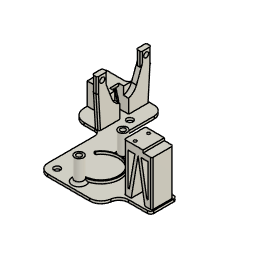
Uchyt na krokovy motor X (Autodesk Fusion 360 design; units mm, degrees)
Autodesk Fusion 360 part; units mm, degrees
sketch "Sketch1" plane through (0, 0, 0) normal (0, 0, 1) x (1, 0, 0)
  line L0 (25, 25) -> (25, -25)
  line L1 (25, -25) -> (-25, -25)
  line L2 (-25, -25) -> (-25, 25)
  circle A0 centre (0, 17.5) radius 2
  circle A1 centre (0, -17.5) radius 2
  line L3 (-48.5, 25) -> (-48.5, 65)
  line L4 (-48.5, 65) -> (-15, 65)
  line L5 (-15, 65) -> (-15, 25)
  line L6 (-25, 25) -> (-48.5, 25)
  line L7 (-15, 25) -> (25, 25)
  line L8 (-48.5, 37.5) -> (-30.5, 37.5)
  line L9 (-30.5, 37.5) -> (-30.5, 52.5)
  line L10 (-30.5, 52.5) -> (-48.5, 52.5)
  line L11 (-48.5, 52.5) -> (-48.5, 37.5)
  line L12 (-30.5, 41.5) -> (-34.5, 41.5)
  line L13 (-34.5, 41.5) -> (-34.5, 48.5)
  line L14 (-34.5, 48.5) -> (-30.5, 48.5)
  line L15 (-30.5, 48.5) -> (-30.5, 41.5)
  line L16 (-30.5, 25) -> (-34.5, 25)
  line L17 (-30.5, 65) -> (-34.5, 65)
  circle A2 centre (0, 17.5) radius 3.5
  circle A3 centre (0, -17.5) radius 3.5
  arc A4 (2.2613, -14.8286) -> (2.2613, 14.8286) centre (0, 0) ccw
  circle A5 centre (8, 0) radius 2.5
  circle A6 centre (-22, 45) radius 2.5
  line L18 (0, 7.5) -> (-12.9904, 7.5)
  line L19 (-12.9904, -7.5) -> (0, -7.5)
  arc A7 (-2.2613, 14.8286) -> (-12.9904, 7.5) centre (0, 0) ccw
  arc A8 (-12.9904, -7.5) -> (-2.2613, -14.8286) centre (0, 0) ccw
  arc A9 (-11.8216, -7.5) -> (-11.8216, 7.5) centre (0, 0) ccw
  dimension "d1" = 50
  dimension "d2" = 50
  dimension "d4" = 4
  dimension "d5" = 4
  dimension "d6" = 17.5
  dimension "d7" = 17.5
  dimension "d12" = 28
  dimension "d57" = 40
  dimension "d62" = 18
  dimension "d63" = 15
  dimension "d64" = 12.5
  dimension "d65" = 4
  dimension "d66" = 7
  dimension "d67" = 4
  dimension "d74" = 7
  dimension "d75" = 7
  dimension "d82" = 5
  dimension "d83" = 8
  dimension "d85" = 17.5
  dimension "d88" = 25
  dimension "d89" = 56.5
  dimension "d91" = 25
  dimension "d167" = 5
  dimension "d220" = 15
  dimension "d221" = 7.5
  constraint horizontal L6
  constraint vertical L0
  constraint horizontal L1
  constraint vertical L2
  constraint coincident A4.centre A7.centre
  constraint vertical L3
  constraint horizontal L4
  constraint vertical L5
  constraint coincident L5.end L6
  constraint collinear L6 L7
  constraint horizontal L8
  constraint vertical L9
  constraint horizontal L10
  constraint vertical L11
  constraint coincident L3 L8.start
  constraint horizontal L12
  constraint vertical L13
  constraint horizontal L14
  constraint vertical L15
  constraint coincident L9 L12.start
  constraint horizontal L16
  constraint coincident L6 L16.start
  constraint horizontal L17
  constraint coincident L4 L17.start
  constraint concentric A0 A2
  constraint coincident A2 A4.end
  constraint coincident A2 A7.start
  constraint concentric A1 A3
  constraint coincident A3 A8.end
  constraint coincident A3 A4.start
  constraint concentric A4 A7
  constraint horizontal L18
  constraint horizontal L19
  constraint concentric A7 A8
  constraint coincident L18 A9.end
  constraint coincident L19 A9.start
  measures "d1" distance of L2.end L0.start
  measures "d2" distance of L2.end L1.end
  measures "d4" diameter of A0
  measures "d5" diameter of A1
  measures "d6" distance of A4.centre A0.centre
  measures "d7" distance of A4.centre A1.centre
  measures "d12" diameter of A9
  measures "d57" distance of L3.start L3.end
  measures "d62" distance of L8.start L8.end
  measures "d63" distance of L8.end L9.end
  measures "d64" distance of L6 L8
  measures "d65" distance of L12.start L12.end
  measures "d66" distance of L12.end L13.end
  measures "d67" distance of L10 L14
  measures "d74" diameter of A2
  measures "d75" diameter of A3
  measures "d82" diameter of A5
  measures "d83" distance of A4.centre A5.centre
  measures "d85" vertical distance of A1.centre A5.centre
  measures "d88" distance of L2 A4.centre
  measures "d89" distance of L3 A5.centre
  measures "d91" vertical distance of L0.end A4.centre
  measures "d167" diameter of A6
  measures "d220" distance of L18.start L19.end
  measures "d221" distance of A4.centre L18
extrude "Extrude1" add sketch "Sketch1" along normal blind 22 contours A0 | A1 makes body 1 at (1.9975, -17.5997, 14.6667) makes body 2 at (1.9975, 17.4003, 14.6667)
extrude "Extrude2" add sketch "Sketch1" along normal blind 2 contours L0 L1 L2 L3 L4 L5 L6 L7 L8 L9 L10 L15 L16 L17 | L3 L8 L9 L10 L11 L12 L13 L14 | L9 L12 L13 L14 L15 | A2 | A2 L18 A7 A9 | A2 A3 A4 A9 | A3 | A3 L19 A8 A9 | A5 | A6 bodies 1 2
extrude "Extrude3" add sketch "Sketch1" along normal blind 4 contours A2 L18 A7 A9 | A2 A3 A4 A9 | A3 L19 A8 A9 bodies 1
extrude "Extrude4" add 2 faces at (0.1483, -18.0912, 22) (-0.1483, 17.7569, 22) along direction (0, 0, 1) blind 2 on bodies 1 bodies 1
fillet "Fillet1" radius 1 2 edges at (-1.8647, -18.2232, 24) (-1.8647, 16.7768, 24) on bodies 1
fillet "Fillet2" radius 0.5 3 edges at (-8.4605, -12.3863, 4) (15, 0, 4) (-8.4605, 12.3863, 4) on bodies 1
sketch "Sketch2" plane through (0, 0, 0) normal (0, 0, 1) x (1, 0, 0)
  line L0 (25, -10.5) -> (50, -10.5)
  line L1 (50, -10.5) -> (50, 10.5)
  line L2 (50, 10.5) -> (25, 10.5)
  line L3 (25, 10.5) -> (25, -10.5)
  line L4 (49, -8.5) -> (27, -8.5)
  line L5 (27, -8.5) -> (27, 8.5)
  line L6 (27, 8.5) -> (49, 8.5)
  line L7 (49, 8.5) -> (49, -8.5)
  dimension "d256" = 1
  constraint horizontal L0
  constraint vertical L1
  constraint horizontal L2
  constraint vertical L3
  constraint horizontal L4
  constraint vertical L5
  constraint horizontal L6
  constraint vertical L7
  measures "d21" distance of L4.start L4.end
  measures "d22" distance of L4.start L6.end
  measures "d23" distance of L0.start L0.end
  measures "d24" distance of L0.end L1.end
  measures "d25" distance of origin L0
  measures "d26" distance of L0 L4
  measures "d27" distance of L1 L7
extrude "Extrude5" add sketch "Sketch2" along normal blind 2 bodies 1
extrude "Extrude6" add sketch "Sketch2" along normal blind 40 contours L4 L5 L6 L7 bodies 1
sketch "Sketch3" plane through (0, 0, 40) normal (0, 0, 1) x (-1, 0, 0)
  line L0 (-49, -8.5) -> (-27, -8.5)
  line L1 (-27, -8.5) -> (-27, 8.5)
  line L2 (-27, 8.5) -> (-49, 8.5)
  line L3 (-49, 8.5) -> (-49, -8.5)
  line L4 (-49, 8.5) -> (-42, 8.5)
  line L5 (-42, 8.5) -> (-42, -8.5)
  line L6 (-42, -8.5) -> (-49, -8.5)
  line L7 (-49, -8.5) -> (-49, 8.5)
  dimension "d32" = 7
  constraint horizontal L4
  constraint vertical L5
  constraint horizontal L6
  constraint vertical L7
  constraint coincident L2.end L3.start
  measures "d32" distance of L2.end L4.end
extrude "Extrude7" cut sketch "Sketch3" against normal blind 2 contours L0 L2 L3 L4 L5 L6 L7 bodies 1
fillet "Fillet3" radius 1 4 edges at (27, 8.5, 21) (27, -8.5, 21) (49, -8.5, 20) (49, 8.5, 20) on bodies 1
sketch "Sketch4" plane through (0, 8.5, 0) normal (0, 1, 0) x (-1, 0, 0)
  line L0 (-48, 38) -> (-48, 2)
  line L1 (-48, 2) -> (-28, 2)
  line L2 (-28, 2) -> (-28, 40)
  line L3 (-28, 40) -> (-42, 40)
  line L4 (-42, 40) -> (-42, 38)
  line L5 (-42, 38) -> (-48, 38)
  line L6 (-43.4614, 2) -> (-38, 34)
  line L7 (-38, 34) -> (-32.538, 2)
  line L8 (-43.4614, 2) -> (-32.538, 2)
  line L9 (-45.9446, 34) -> (-40.5, 34)
  line L10 (-40.5, 34) -> (-44.9517, 7.9159)
  line L11 (-45.9446, 8) -> (-45.9446, 34)
  line L12 (-35.5, 34) -> (-30.0549, 34)
  line L13 (-30.0549, 34) -> (-30.0549, 8)
  line L14 (-31.0478, 7.9159) -> (-35.5, 34)
  arc A0 (-45.9446, 8) -> (-44.9517, 7.9159) centre (-45.4446, 8) ccw
  arc A1 (-31.0478, 7.9159) -> (-30.0549, 8) centre (-30.5549, 8) ccw
  dimension "d42" = 0.5
  dimension "d43" = 0.5
  dimension "d44" = 6
  dimension "d45" = 6
  dimension "d239" = 10
  dimension "d241" = 2.5
  dimension "d242" = 2.5
  dimension "d247" = 32
  dimension "d248" = 32
  dimension "d249" = 32
  constraint coincident L1 L6.start
  constraint coincident L1 L7.end
  constraint parallel L6 L10
  constraint perpendicular L9 L11
  constraint perpendicular L11 L12
  constraint perpendicular L12 L13
  constraint tangent L10 A0
  constraint tangent L11 A0
  constraint tangent L13 A1
  constraint tangent L14 A1
  constraint parallel L7 L14
  constraint parallel L8 L9
  measures "d42" radius of A0
  measures "d43" radius of A1
  measures "d44" distance of L8 A0.centre
  measures "d45" distance of L1 A1.centre
  measures "d239" distance of L2 L6.end
  measures "d241" horizontal distance of L6.end L9.end
  measures "d242" horizontal distance of L6.end L12.start
  measures "d247" distance of L8 L9
  measures "d248" distance of L8 L12
  measures "d249" distance of L6.end L8
extrude "Extrude8" cut sketch "Sketch4" against normal up to surface (17 mm away) contours L1 L6 L7 L8 bodies 1
extrude "Extrude9" cut sketch "Sketch4" against normal up to surface (17 mm away) contours L9 L10 L11 A0 | L12 L13 L14 A1 bodies 1
sketch "Sketch6" plane through (0, 0, 0) normal (0, 0, -1) x (1, 0, 0)
  line L0 (25, 25) -> (-25, 25)
  line L1 (-25, 25) -> (-25, -25)
  line L2 (-15, -25) -> (25, -25)
  line L3 (25, -25) -> (25, -10.5)
  circle A0 centre (38, 0) radius 2.5
  circle A1 centre (17.5, -17.5) radius 2.5
  line L4 (25, -25) -> (25, 25)
  circle A2 centre (-17.5, 17.5) radius 2.5
  line L5 (25, 25) -> (-25, 25)
  line L6 (-25, 25) -> (-25, -25)
  line L7 (-15, -65) -> (-15, -25)
  line L8 (-25, -25) -> (-48.5, -25)
  line L9 (-48.5, -25) -> (-48.5, -65)
  line L10 (-48.5, -65) -> (-15, -65)
  line L11 (-25, -25) -> (-48.5, -25)
  line L12 (25, -10.5) -> (50, -10.5)
  line L13 (50, -10.5) -> (50, 10.5)
  line L14 (50, 10.5) -> (25, 10.5)
  line L15 (25, 10.5) -> (25, 25)
  dimension "d46" = 5
  dimension "d47" = 5
  dimension "d48" = 7.5
  dimension "d50" = 5
  dimension "d51" = 7.5
  dimension "d52" = 7.5
  measures "d46" diameter of A0
  measures "d47" diameter of A1
  measures "d48" distance of A1.centre L4
  measures "d50" diameter of A2
  measures "d51" distance of A2.centre L5
  measures "d52" distance of A2.centre L6
extrude "Extrude10" cut sketch "Sketch6" against normal up to surface (2 mm away) contours A0 | A1 | A2 bodies 1
extrude "Extrude11" add sketch "Sketch1" along normal up to surface (4 mm away) contours A2 A3 A4 A9 bodies 1
extrude "Extrude12" add sketch "Sketch1" along normal blind 20 contours A2 | A3 bodies 1
extrude "Extrude13" cut sketch "Sketch1" along normal up to surface (24 mm away) contours A0 | A1 bodies 1
extrude "Extrude14" add sketch "Sketch1" along normal blind 18.5 contours L3 L8 L9 L10 L11 L12 L13 L14 bodies 1
extrude "Extrude15" add 1 faces at (-43.8333, 46.1667, 18.5) along direction (0, 0, 1) blind 2 on bodies 1 bodies 1
extrude "Extrude17" cut sketch "Sketch1" along normal blind 2 contours A6 bodies 1
sketch "Sketch7" plane through (-48.5, 0, 0) normal (-1, 0, 0) x (0, -1, 0)
  line L0 (-65, 0) -> (-25, 0)
  line L1 (-48.5, 2.5) -> (-45.3117, 17.5)
  line L2 (-45.3117, 17.5) -> (-44.6883, 17.5)
  line L3 (-44.6883, 17.5) -> (-41.5, 2.5)
  line L4 (-41.5, 2.5) -> (-48.5, 2.5)
  line L5 (-52.5, 20.5) -> (-52.5, 2)
  line L6 (-37.5, 2) -> (-37.5, 20.5)
  line L7 (-48.5, 17.5) -> (-46.334, 17.5)
  line L8 (-46.334, 17.5) -> (-48.5, 7.3097)
  line L9 (-48.5, 17.5) -> (-48.5, 7.3097)
  line L10 (-41.5, 17.5) -> (-43.666, 17.5)
  line L11 (-43.666, 17.5) -> (-41.5, 7.3097)
  line L12 (-41.5, 17.5) -> (-41.5, 7.3097)
  line L13 (-25, 2) -> (-37.5, 2)
  line L14 (-37.5, 20.5) -> (-52.5, 20.5)
  line L15 (-52.5, 2) -> (-65, 2)
  line L16 (-65, 2) -> (-65, 0)
  line L17 (-25, 0) -> (-25, 2)
  line L18 (-37.5, 2) -> (-37.5, 20.5)
  line L19 (-52.5, 20.5) -> (-52.5, 2)
  dimension "d142" = 78
  dimension "d143" = 78
  dimension "d144" = 4
  dimension "d145" = 4
  dimension "d147" = 4
  dimension "d149" = 1
  dimension "d150" = 78
  dimension "d152" = 1
  dimension "d153" = 4
  constraint perpendicular L7 L9
  measures "d142" angle of L3 L4
  measures "d143" angle of L1 L4
  measures "d144" distance of L1.start L5
  measures "d145" distance of L3.end L6
  measures "d147" distance of L5 L7.start
  measures "d149" distance of L1 L8.end
  measures "d150" angle of L7 L8
  measures "d152" distance of L3 L11
  measures "d153" distance of L6 L12
extrude "Extrude18" cut sketch "Sketch7" against normal up to surface (14 mm away) contours L1 L2 L3 L4 | L7 L8 L9 | L10 L11 L12 bodies 1
sketch "Sketch9" plane through (-30.5, 0, 0) normal (1, 0, 0) x (0, 1, 0)
  line L0 (37.5, 2) -> (41.5, 2)
  line L1 (41.5, 20.5) -> (37.5, 20.5)
  line L2 (25.1524, 0) -> (41.5, 0)
  line L3 (41.5, 0) -> (41.5, 13.0164)
  line L4 (23.5, 27.99) -> (23.5, 40)
  line L5 (23.5, 40) -> (31.5, 40)
  line L6 (31.5, 40) -> (31.5, 28.9965)
  line L7 (23.5, 27.99) -> (25.1524, 0)
  line L8 (37.5, 13.0164) -> (41.5, 13.0164)
  circle A0 centre (27.5, 36) radius 2
  line L9 (31.5, 28.9965) -> (37.5, 13.0164)
  line L10 (45, 2) -> (45, 38)
  line L11 (48.5, 0) -> (48.5, 13.0164)
  line L12 (58.5, 40) -> (58.5, 28.9965)
  line L13 (66.5, 40) -> (58.5, 40)
  line L14 (66.5, 27.99) -> (66.5, 40)
  circle A1 centre (62.5, 36) radius 2
  line L15 (66.5, 27.99) -> (64.8476, 0)
  line L16 (64.8476, 0) -> (48.5, 0)
  line L17 (41.5, 2) -> (41.5, 20.5)
  line L18 (48.5, 13.0164) -> (52.5, 13.0164)
  line L19 (52.5, 13.0164) -> (58.5, 28.9965)
  line L20 (52.5, 2) -> (52.5, 20.5)
  dimension "d170" = 36
  dimension "d171" = 4
  dimension "d172" = 4
  dimension "d173" = 4
  dimension "d176" = 17.5
  dimension "d217" = 11.0035
  dimension "d218" = 40
  dimension "d219" = 4
  constraint horizontal L2
  constraint vertical L3
  constraint vertical L4
  constraint horizontal L5
  constraint vertical L6
  constraint perpendicular L3 L8
  constraint symmetric L2.start L10 L15.end
  constraint symmetric L2.end L10 L11.start
  constraint symmetric L3.end L10 L11.end
  constraint symmetric L4.start L10 L14.start
  constraint symmetric L4.end L10 L13.start
  constraint symmetric L5.end L10 L12.start
  constraint symmetric A0 L10 A1
  constraint symmetric L6.end L10 L12.end
  constraint coincident L3.end L17
  constraint perpendicular L11 L18
  constraint coincident L18.end L20
  measures "d170" distance of L2 A0.centre
  measures "d171" distance of L5 A0.centre
  measures "d172" distance of L6 A0.centre
  measures "d173" distance of L4 A0.centre
  measures "d176" horizontal distance of A0.centre L10.end
  measures "d217" distance of L5.end L6.end
  measures "d218" distance of origin L5
  measures "d219" diameter of A0
extrude "Extrude20" add sketch "Sketch9" along normal blind 4 bodies 1
fillet "Fillet27" radius 11 1 edges at (25, 10.5, 1) on bodies 1
fillet "Fillet28" radius 12 1 edges at (25, 25, 1) on bodies 1
fillet "Fillet29" radius 12 1 edges at (-15, 25, 1) on bodies 1
fillet "Fillet30" radius 7.5 1 edges at (-15, 65, 1) on bodies 1
fillet "Fillet31" radius 8 1 edges at (-48.5, 65, 1) on bodies 1
fillet "Fillet32" radius 10 1 edges at (-48.5, 25, 1) on bodies 1
fillet "Fillet33" radius 5 1 edges at (-25, 25, 1) on bodies 1
fillet "Fillet34" radius 7.5 1 edges at (-25, -25, 1) on bodies 1
fillet "Fillet35" radius 9 1 edges at (25, -25, 1) on bodies 1
fillet "Fillet36" radius 7.5 1 edges at (25, -10.5, 1) on bodies 1
fillet "Fillet37" radius 2.5 1 edges at (50, -10.5, 1) on bodies 1
fillet "Fillet38" radius 2.5 1 edges at (50, 10.5, 1) on bodies 1
fillet "Fillet39" radius 1 8 edges at (-30.5, 65.7328, 14.995) (-26.5, 65.7328, 14.995) (-30.5, 24.2672, 14.995) (-26.5, 24.2672, 14.995) (-26.5, 23.5, 33.995) (-30.5, 23.5, 33.995) (-26.5, 66.5, 33.995) (-30.5, 66.5, 33.995) on bodies 1
fillet "Fillet44" radius 1 4 edges at (-26.5, 31.5, 34.4983) (-30.5, 31.5, 34.4983) (-26.5, 58.5, 34.4983) (-30.5, 58.5, 34.4983) on bodies 1
extrude "Extrude21" cut 1 faces at (-43.8333, 46.1667, 20.5) along direction (0, 0, -1) blind 0.984 on bodies 1 bodies 1
fillet "Fillet45" radius 2 2 edges at (0, 21, 2) (0, -21, 2) on bodies 1
sketch "Sketch11" plane through (0, 0, 40) normal (0, 0, 1) x (-1, 0, 0)
  arc A0 (-27, 7.5) -> (-28, 8.5) centre (-28, 7.5) ccw
  line L0 (-28, 8.5) -> (-42, 8.5)
  line L1 (-42, 8.5) -> (-42, -8.5)
  line L2 (-42, -8.5) -> (-28, -8.5)
  arc A1 (-28, -8.5) -> (-27, -7.5) centre (-28, -7.5) ccw
  line L3 (-27, -7.5) -> (-27, 7.5)
  circle A2 centre (-32.6, 5.34) radius 1.15
  circle A3 centre (-32.6, -5.34) radius 1.15
  dimension "d230" = 2.3
  dimension "d231" = 5.6
  dimension "d232" = 3.16
  dimension "d235" = 0
  dimension "d236" = -10.68
  measures "d230" diameter of A2
  measures "d231" distance of L3 A2.centre
  measures "d232" distance of L0 A2.centre
extrude "Extrude23" cut sketch "Sketch11" against normal blind 5.8 contours A2 | A3 bodies 1
fillet "Fillet47" radius 3.5 2 edges at (-30.5, 37.5, 7.5082) (-30.5, 52.5, 7.5082) on bodies 1
fillet "Fillet48" radius 10 2 edges at (-28.5, 37.5, 13.0164) (-28.5, 52.5, 13.0164) on bodies 1
chamfer "Chamfer1" distance 1 angle 45 2 edges at (-1.8647, -18.2232, 0) (-1.8647, 16.7768, 0) on bodies 1
